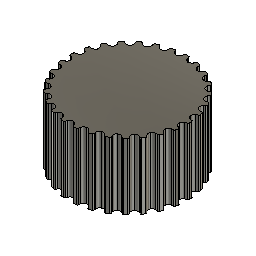
gear_29z (Autodesk Fusion 360 design; units mm, degrees)
Autodesk Fusion 360 part; units mm, degrees
sketch "Sketch1" plane through (0, 0, 0) normal (0, 0, 1) x (1, 0, 0) in component "gt2 pulley"
  circle A0 centre (0, 0) radius 9.231 construction
  circle A1 centre (0, 0) radius 8.227 construction
  line L0 (0, 0) -> (0, 9.231) construction
  line L1 (0, 0) -> (0.998, 9.1769) construction
  line L2 (0, 0) -> (1.4103, 9.1226) construction
  circle A2 centre (0, 0) radius 8.977 construction
  arc A3 (0.3724, 8.8304) -> (0.4231, 8.5545) centre (1.3715, 8.8716) ccw
  circle A4 centre (0, 0) radius 8.827 construction
  arc A5 (0.2262, 8.9741) -> (0, 8.977) centre (0, 0) ccw
  arc A6 (0.3724, 8.8304) -> (0.2262, 8.9741) centre (0.2225, 8.8242) ccw
  arc A7 (0.4231, 8.5545) -> (0.8895, 8.1788) centre (0.9495, 8.7305) ccw
  arc A8 (0, 8.977) -> (-0.2262, 8.9741) centre (0, 0) ccw
  arc A9 (-0.2262, 8.9741) -> (-0.3724, 8.8304) centre (-0.2225, 8.8242) ccw
  arc A10 (-0.4231, 8.5545) -> (-0.3724, 8.8304) centre (-1.3715, 8.8716) ccw
  arc A11 (-0.8895, 8.1788) -> (-0.4231, 8.5545) centre (-0.9495, 8.7305) ccw
  arc A12 (0.8895, 8.1788) -> (-0.8895, 8.1788) centre (0, 0) ccw
  point P0 (1.3715, 8.8716)
  point P1 (0, 8.977)
  dimension "d18" = 18.462
  dimension "d19" = 6.207
  dimension "d22" = 1.004
  dimension "d24" = 0.75
  dimension "d26" = 1
  dimension "d27" = 0.15
  dimension "d28" = 0.15
  dimension "d47" = 0.555
  dimension "d52" = 3.812
  constraint coincident A0.centre A1.centre
  constraint coincident A0 L0.end
  constraint vertical L0
  constraint coincident A0 L1.end
  constraint coincident A0 L2.end
  constraint concentric A1 A2
  constraint coincident A1 A7.end
  constraint coincident L1 A7.end
  constraint coincident A2 P0
  constraint coincident L2 P0
  constraint coincident P0 A3.centre
  constraint coincident A2 P1
  constraint coincident L0 P1
  constraint concentric A2 A4
  constraint coincident P1 A5.end
  constraint coincident A4 A6.centre
  constraint coincident A3.start A6.start
  constraint tangent A3 A6
  constraint tangent A3 A7
  constraint symmetric L0 A7.end A11.start
  constraint symmetric L0 A3.start A9.end
  constraint symmetric L0 A3.end A10.start
  constraint symmetric L0 A3 A10
  constraint symmetric L0 A5.start A8.end
  constraint symmetric L0 P1 A5.end
  constraint symmetric L0 A5 A8
  constraint symmetric L0 A6 A9
  constraint symmetric L0 A7 A11
  constraint coincident A1 A11.start
  constraint tangent A1 A7
  constraint coincident L1 A7.centre
  measures "d18" diameter of A0
  measures "d19" angle of L0 L1
  measures "d22" distance of A0 A1
  measures "d24" distance of A1 A2
  measures "d26" radius of A3
  measures "d27" distance of A2 A4
  measures "d28" radius of A6
  measures "d47" radius of A7
extrude "Extrude1" add sketch "Sketch1" along normal blind 10 makes body 1
pattern_circular "C-Pattern1" count 29 over 360 about axis through (0, 0, 1.75) along (0, 0, 1) of bodies 1 makes body 2 at (-2.4385, 7.8573, 6.6667) makes body 3 at (-4.0706, 7.1494, 6.6667) makes body 4 at (-4.4099, 6.9452, 3.3333) makes body 5 at (-6.334, 5.2502, 6.6667) makes body 6 at (-7.5672, 3.2282, 6.6667) makes body 7 at (-7.7138, 2.8603, 3.3333) makes body 8 at (-8.2233, -0.2475, 6.6667) makes body 9 at (-8.102, -1.4286, 6.6667) makes body 10 at (-7.8718, -2.3911, 3.3333) makes body 11 at (-6.3967, -5.1736, 6.6667) makes body 12 at (-5.135, -6.4277, 6.6667) makes body 13 at (-3.6331, -7.3813, 6.6667) makes body 14 at (-1.9614, -7.9897, 6.6667) makes body 15 at (-0.198, -8.2246, 6.6667) makes body 16 at (1.5747, -8.0749, 6.6667) makes body 17 at (3.2737, -7.5476, 6.6667) makes body 18 at (4.8197, -6.6674, 6.6667) makes body 19 at (5.7292, -5.9042, 6.6667) makes body 20 at (6.8645, -4.5346, 6.6667) makes body 21 at (7.3593, -3.6775, 3.3333) makes body 22 at (7.9778, -2.0095, 3.3333) makes body 23 at (8.1483, 1.1352, 6.6667) makes body 24 at (7.7138, 2.8603, 6.6667) makes body 25 at (7.5672, 3.2282, 3.3333) makes body 26 at (5.7998, 5.8348, 6.6667) makes body 27 at (4.4099, 6.9452, 6.6667) makes body 28 at (2.8138, 7.7308, 6.6667) makes body 29 at (1.6717, 8.0554, 6.6667)
sketch "Sketch2" plane through (0, 0, 10) normal (0, 0, 1) x (-1, 0, 0)
  arc A0 (-6.9713, -5.4328) -> (-6.9862, -5.6373) centre (-6.8695, -5.5431) ccw
  arc A1 (-6.9862, -5.6373) -> (-6.6933, -5.9822) centre (0, 0) ccw
  arc A2 (-6.6933, -5.9822) -> (-6.4891, -6.0005) centre (-6.5814, -5.8823) ccw
  arc A3 (-6.246, -5.8606) -> (-6.4891, -6.0005) centre (-5.8737, -6.7887) ccw
  arc A4 (-5.6577, -5.9728) -> (-6.246, -5.8606) centre (-6.0394, -6.3757) ccw
  arc A5 (-6.8094, -4.6169) -> (-5.6577, -5.9728) centre (0, 0) ccw
  arc A6 (-6.7939, -5.2156) -> (-6.8094, -4.6169) centre (-7.2688, -4.9283) ccw
  arc A7 (-6.9713, -5.4328) -> (-6.7939, -5.2156) centre (-7.6495, -4.698) ccw
  circle A8 centre (0, 0) radius 8.227
  constraint concentric A1 A8
extrude "Extrude2" add sketch "Sketch2" against normal blind 10 contours A5 A8 bodies 1 2 3 4 5 6 7 8 9 10 11 12 13 14 15 16 17 18 19 20 21 22 23 24 25 26 27 28 29
extrude "Extrude4" [suppressed] in component "gt2 pulley"
pattern_circular "C-Pattern7" [suppressed] in component "gt2 pulley"
extrude "Extrude3" [suppressed] in component "gt2 pulley"
pattern_circular "C-Pattern6" [suppressed] in component "gt2 pulley"
extrude "Extrude2'" [suppressed] in component "gt2 pulley"
pattern_circular "C-Pattern5" [suppressed] in component "gt2 pulley"
extrude "Extrude1'" [suppressed] in component "gt2 pulley"
pattern_circular "C-Pattern4" [suppressed] in component "gt2 pulley"
pattern_circular "C-Pattern3" [suppressed] in component "gt2 pulley"
pattern_circular "C-Pattern2" [suppressed] in component "gt2 pulley"
pattern_circular "C-Pattern1'" [suppressed] in component "gt2 pulley"
copy_body "Body->Comp1" [suppressed] in component "Component"
copy_body "Body->Comp2" [suppressed] in component "Component'"
copy_body "Body->Comp3" [suppressed] in component "Component''"
copy_body "Body->Comp4" [suppressed] in component "Component'''"
copy_body "Body->Comp5" [suppressed] in component "Component''''"
copy_body "Body->Comp6" [suppressed] in component "Component'''''"
copy_body "Body->Comp7" [suppressed] in component "Component''''''"
copy_body "Body->Comp8" [suppressed] in component "Component'''''''"
copy_body "Body->Comp9" [suppressed] in component "Component''''''''"
copy_body "Body->Comp10" [suppressed] in component "Component'''''''''"
copy_body "Body->Comp11" [suppressed] in component "Component''''''''''"
copy_body "Body->Comp12" [suppressed] in component "Component'''''''''''"
copy_body "Body->Comp13" [suppressed] in component "Component''''''''''''"
copy_body "Body->Comp14" [suppressed] in component "Component'''''''''''''"
copy_body "Body->Comp15" [suppressed] in component "Component''''''''''''''"
copy_body "Body->Comp16" [suppressed] in component "Component'''''''''''''''"
copy_body "Body->Comp17" [suppressed] in component "Component''''''''''''''''"
copy_body "Body->Comp18" [suppressed] in component "Component'''''''''''''''''"
copy_body "Body->Comp19" [suppressed] in component "Component''''''''''''''''''"
copy_body "Body->Comp20" [suppressed] in component "Component'''''''''''''''''''"
component "gt2 pulley" placed x (1, 0, 0) y (0, 1, 0) z (0, 0, 1) at (0, 0, 0)
equation "NumTeeth = 29" comment "min 20"
equation "ToothPitch = 2 mm"
equation "PullyDia = NumTeeth * ToothPitch / PI"
equation "ToothAng = ( ( 360 / NumTeeth ) * 1 deg )"
equation "TransOffsetAngle = ToothAng * 0.2"
equation "Sholulder_Radius = 0.15 mm"
equation "Root_Radius = 0.555 mm"
equation "TransRadius = 1 mm"
equation "ToolHeight = 0.75 mm"
equation "PLD = 0.254 mm"
equation "d18 = PullyDia"
equation "d19 = ToothAng / 2"
equation "d22 = PLD + ToolHeight"
equation "d24 = ToolHeight"
equation "d26 = TransRadius"
equation "d27 = Sholulder_Radius"
equation "d31 = NumTeeth"
equation "d33 = NumTeeth"
equation "d35 = NumTeeth"
equation "d37 = NumTeeth"
equation "d41 = NumTeeth"
equation "d45 = NumTeeth"
equation "d47 = Root_Radius"
equation "d50 = NumTeeth"
